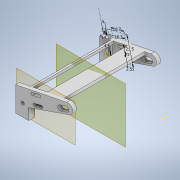
# Autodesk Inventor part: Capping_RotatingArm
Saved by Autodesk Inventor 2022 (Build 260153000, 153)
## iProperties
Created: 2024-05-06
Part Number: Capping_RotatingArm
Material: Generic
Document SubType Name: Modeling
Designer: Gotham City
Density: 1 g/cm^3
Appearance: Default
Author: Gotham City
Autodesk Inventor part; units mm, degrees
ref_plane "YZ Plane" through (0, 0, 0) normal (1, 0, 0) x (0, 1, 0)
ref_plane "XZ Plane" through (0, 0, 0) normal (0, 1, 0) x (-1, 0, 0)
ref_plane "XY Plane" through (0, 0, 0) normal (0, 0, 1) x (1, 0, 0)
sketch "Sketch1" plane through (0, 0, 0) normal (0, 0, 1) x (1, 0, 0)
  line L0 (-13.4159, 40.4526) -> (-44.6613, 29.6117) construction
  circle A0 centre (-45.1029, 22.9379) radius 1.3 projected
  line L1 (-41.8029, 32.9379) -> (-41.8029, 12.9379) projected
  line L2 (-11.7769, 35.7289) -> (-42.4029, 25.1029) construction
  point P0 (0, 0)
sketch "Sketch3" plane through (0, 0, 0) normal (0, 0, 1) x (1, 0, 0)
  line L0 (-41.8029, 32.9379) -> (-41.8029, 12.9379) construction
  line L1 (-41.8029, 12.9379) -> (-50.8029, 12.9379)
  line L2 (-50.8029, 12.9379) -> (-50.8029, 32.9379)
  line L3 (-50.8029, 32.9379) -> (-41.8029, 32.9379)
  line L4 (-41.8029, 32.9379) -> (-41.8029, 12.9379)
  line L5 (-50.8029, 22.9379) -> (-41.8029, 22.9379) construction
  circle A0 centre (-45.1029, 22.9379) radius 1.3 projected
  line L6 (-13.4159, 40.4526) -> (-44.5892, 29.6368)
  line L7 (-44.5892, 29.6368) -> (-41.8029, 21.6064)
  line L8 (-41.8029, 21.6064) -> (-10.6297, 32.4223)
  line L9 (-10.6297, 32.4223) -> (-13.4159, 40.4526)
  line L10 (-13.4159, 40.4526) -> (-41.8029, 21.6064) construction
  line L11 (-44.5892, 29.6368) -> (-10.6297, 32.4223) construction
  line L12 (-42.4029, 25.1029) -> (-11.7769, 35.7289) construction
  line L13 (-13.4159, 40.4526) -> (-44.6613, 29.6117) construction
  circle A1 centre (-11.7769, 35.7289) radius 1.5 construction
  line L14 (-50.8029, 32.9379) -> (-13.4159, 40.4526)
  line L15 (-13.4159, 40.4526) -> (-9.411, 41.2576)
  line L16 (-11.7769, 35.7289) -> (-9.8874, 36.3845) construction
  line L17 (-13.9556, 32.856) -> (-9.2319, 34.495)
  line L18 (-10.543, 38.274) -> (-15.2668, 36.635)
  arc A2 (-9.2319, 34.495) -> (-10.543, 38.274) centre (-9.8874, 36.3845) ccw
  line L19 (-10.6297, 32.4223) -> (-7.3157, 33.5721)
  arc A3 (-7.3157, 33.5721) -> (-9.411, 41.2576) centre (-8.6243, 37.3437) ccw
  arc A4 (-15.2668, 36.635) -> (-13.9556, 32.856) centre (-14.6112, 34.7455) ccw
  point P0 (0, 0)
  point P1 (-27.6094, 31.0295)
  point P2 (-41.8029, 30.6035)
  point P3 (-11.2853, 34.3118)
  point P4 (-12.2686, 37.146)
  point P5 (-10.8322, 36.0567)
  dimension "d0" = 9
  dimension "d1" = 3.5
  dimension "d2" = 0
  dimension "d3" = 3
  dimension "d45" = 4
  dimension "d46" = 2
  dimension "d48" = 7.5
  dimension "d65" = 3
  constraints: 39 end point, 6 parallel, 6 point on circle, 6 tangent, 5 midpoint, 5 point on line, 4 centre point, 3 coincident, 3 perpendicular, 2 collinear, 1 horizontal
  measures "d0" distance of L2.end L3.end
  measures "d1" distance between parallel lines of L8 L12
  measures "d2" distance between parallel lines of L6 L13
  measures "d3" diameter of A1
  measures "d45" distance between parallel lines of L17 L18
  measures "d46" distance of L16.start L16.end
  measures "d65" distance of A4.centre L12.end
extrude "Extrusion1" add sketch "Sketch3" against normal blind 3 contours L1 L2 L3 L4 L6 L7 | L7 L6 L4 | L4 L6 L9 L18 A4 L17 L8 | L14 L6 L4 L3 | L9 L17 A2 L18 L15 A3 L19
ref_plane "Work Plane2" through (0, 0, 32.5) normal (0, 0, 1) x (1, 0, 0)
ref_plane "Work Plane1" through (0, 0, 65) normal (0, 0, 1) x (1, 0, 0)
sketch "Sketch12" plane through (0, 0, -3) normal (0, 0, 1) x (1, 0, 0)
  line L0 (-41.8029, 21.6064) -> (-41.8029, 12.9379) projected
  line L1 (-41.8029, 12.9379) -> (-41.8029, 34.7469)
  line L2 (-41.8029, 34.7469) -> (-40.3029, 35.0484)
  line L3 (-40.3029, 35.0484) -> (-40.3029, 12.9379)
  line L4 (-40.3029, 12.9379) -> (-41.8029, 12.9379)
  line L5 (-9.411, 41.2576) -> (-50.8029, 32.9379) projected
  point P0 (0, 0)
  dimension "d50" = 1.5
  constraints: 8 end point, 2 point on line, 1 collinear, 1 parallel, 1 perpendicular
  measures "d50" distance between parallel lines of L3 L0
extrude "Extrusion9" add sketch "Sketch12" along normal blind 5
thicken "Thicken3" operation add thickness 0.1 both sides no extend neighbours yes toward (1, 0, 0) faces at (-41.8029, 27.4772, 1.3333)
mirror "Mirror1" about plane through (0, 0, 32.5) normal (0, 0, 1) of "Extrusion1", "Extrusion9", "Thicken3"
sketch "Sketch4" plane through (0, 0, 0) normal (0, 0, 1) x (1, 0, 0)
  line L0 (-14.4375, 40.2473) -> (-13.7819, 38.3578)
  line L1 (-13.4159, 40.4526) -> (-44.6613, 29.6117) construction
  line L2 (-13.7819, 38.3578) -> (-27.0084, 33.7687)
  line L3 (-27.0084, 33.7687) -> (-28.2902, 37.4629)
  line L4 (-13.4159, 40.4526) -> (-28.2902, 37.4629)
  line L5 (-50.8029, 32.9379) -> (-9.411, 41.2576) projected
  point P0 (0, 0)
  point P1 (-14.4375, 40.2473)
  point P2 (-14.4375, 40.2473)
  dimension "d8" = 2
  dimension "d9" = 14
  constraints: 6 end point, 2 point on line, 1 perpendicular, 5 other
  measures "d8" distance of point (-14.437, 40.247) L2.start
  measures "d9" distance of L2.start L2.end
extrude "Extrusion2" add sketch "Sketch4" along normal up to surface (65 mm away)
sketch "Sketch10" plane through (-27.0084, 33.7687, 0) normal (0.3277907, -0.9447504, 0) x (0.9447504, 0.3277907, 0)
  line L0 (14, 0) -> (14, 65) construction
  line L1 (0, 0) -> (0, 65) construction
  circle A0 centre (6, 14.5) radius 5
  line L2 (-50.9309, 32.5) -> (44.3132, 32.5) projected
  point P0 (14.4471, 0)
  point P1 (5.5291, 32.5)
  dimension "d25" = 10
  dimension "d28" = 8
  dimension "d68" = 18
  constraints: 1 centre point, 1 point on line
  measures "d25" diameter of A0
  measures "d28" distance from line of A0.centre L0
  measures "d68" vertical distance of A0.centre point (5.529, 32.5)
extrude "Extrusion8" cut sketch "Sketch10" against normal blind 2
draft "FaceDraft1" angle 2.5 pull direction (-0.3277907, 0.9447504, 0) faces at (-17.069, 38.63, 14.0977) fixed edges at (-26.7199, 35.9879, 14.5)
sketch "Sketch16" plane through (0, 0, 0) normal (0, 0, 1) x (1, 0, 0)
  line L0 (-50.8029, 32.9379) -> (-9.411, 41.2576) projected
  line L1 (-39.7029, 35.169) -> (-39.7029, 33.129)
  line L2 (-39.7029, 33.129) -> (-41.7029, 32.727)
  line L3 (-41.7029, 34.767) -> (-41.7029, 12.9379) projected
  line L4 (-41.7029, 34.767) -> (-39.7029, 35.169)
  line L5 (-28.2902, 37.4629) -> (-40.3029, 35.0484) projected
  line L6 (-50.8029, 32.9379) -> (-9.411, 41.2576) projected
  line L7 (-41.7029, 32.727) -> (-41.7029, 34.767)
  point P0 (0, 0)
  dimension "d61" = 2
  dimension "d62" = 2
  constraints: 8 end point, 2 collinear, 2 point on line, 1 parallel, 1 vertical
  measures "d61" distance between parallel lines of L0 L2
  measures "d62" distance between parallel lines of L3 L1
extrude "Extrusion12" add sketch "Sketch16" along normal up to surface (65 mm away)
mirror "Mirror2" about plane through (0, 0, 32.5) normal (0, 0, 1) of "Extrusion8", "FaceDraft1"
sketch "Sketch18" plane through (0, 0, -3) normal (0, 0, -1) x (-1, 0, 0)
  circle A0 centre (32.8063, 27.1171) radius 1 construction
  line L0 (50.8029, 12.9379) -> (50.8029, 32.9379) construction
  circle A1 centre (34.5371, 33.8998) radius 1 construction
  circle A2 centre (45.1029, 22.9379) radius 1.3 construction
  circle A3 centre (45.1029, 22.9379) radius 2.25 construction
  line L1 (28.5428, 20.7228) -> (33.859, 41.5552) construction
  line L2 (33.859, 41.5552) -> (44.2267, 38.9094) construction
  line L3 (44.2267, 38.9094) -> (38.9105, 18.0771) construction
  line L4 (38.9105, 18.0771) -> (28.5428, 20.7228) construction
  line L5 (54.7994, 49.604) -> (46.0227, 15.2108) construction
  line L6 (34.5371, 33.8998) -> (32.8063, 27.1171) construction
  line L7 (31.2009, 31.139) -> (41.5686, 28.4932) construction
  circle A4 centre (48.3029, 34.2571) radius 2.5 construction
  line L8 (32.8063, 27.1171) -> (32.2462, 24.9222) construction
  line L9 (40.3029, 22.1268) -> (7.3157, 33.5721) construction
  line L10 (34.5371, 33.8998) -> (35.0973, 36.0947) construction
  line L11 (28.2902, 37.4629) -> (39.7029, 35.169) construction
  point P0 (0, 0)
  point P1 (33.6717, 30.5085)
  dimension "d69" = 2
  dimension "d71" = 7
  dimension "d78" = 4.5
  dimension "d79" = 14.316
  dimension "d80" = 21.5
  dimension "d82" = 10.7
  dimension "d83" = 18.3
  dimension "d84" = 2.55
  dimension "d85" = 5
  dimension "d86" = 3.5
  constraints: 18 end point, 4 centre point, 4 parallel, 4 point on line, 3 midpoint, 2 collinear, 2 tangent, 1 coincident, 1 equal radius, 1 perpendicular
  measures "d69" diameter of A0
  measures "d71" distance of L6.start L6.end
  measures "d78" diameter of A3
  measures "d79" angle of L0 L5
  measures "d80" distance of L1.start L1.end
  measures "d82" distance of L1.end L2.end
  measures "d83" distance between parallel lines of L1 L5
  measures "d84" distance from line of L1 L6.end
  measures "d85" diameter of A4
  measures "d86" distance from line of L2 A4.centre
sketch "Sketch19" plane through (0, 0, -3) normal (0, 0, -1) x (-1, 0, 0)
  line L0 (35.7131, 26.3753) -> (29.8994, 27.8589) construction
  line L1 (35.4659, 25.4064) -> (29.6522, 26.89)
  line L2 (30.1467, 28.8279) -> (35.9604, 27.3443)
  arc A0 (35.4659, 25.4064) -> (35.9604, 27.3443) centre (35.7131, 26.3753) ccw
  arc A1 (30.1467, 28.8279) -> (29.6522, 26.89) centre (29.8994, 27.8589) ccw
  line L3 (34.5371, 33.8998) -> (32.8063, 27.1171) construction
  line L4 (31.2009, 31.139) -> (41.5686, 28.4932) construction
  line L5 (37.444, 33.158) -> (31.6303, 34.6416) construction
  line L6 (37.6912, 34.1269) -> (31.8776, 35.6105)
  line L7 (31.383, 33.6726) -> (37.1967, 32.189)
  arc A2 (37.1967, 32.189) -> (37.6912, 34.1269) centre (37.444, 33.158) ccw
  arc A3 (31.8776, 35.6105) -> (31.383, 33.6726) centre (31.6303, 34.6416) ccw
  point P0 (0, 0)
  dimension "d87" = 2
  dimension "d88" = 6
  dimension "d53" = 1
  constraints: 16 end point, 8 point on circle, 6 symmetric about line, 4 centre point, 4 tangent, 1 midpoint, 1 parallel, 1 perpendicular, 2 other
  measures "d87" distance between parallel lines of L2 L1
  measures "d88" distance of L0.start L0.end
extrude "Extrusion13" cut sketch "Sketch19" against normal up to surface (71 mm away)
sketch "Sketch15" plane through (-41.8029, 12.9379, 65) normal (-1, 0, 0) x (0, 0, 1)
  line L0 (-49.115, 0) -> (-49.115, 17.165) construction
  line L1 (-49.115, 17.165) -> (-16.115, 17.165) construction
  line L2 (-16.115, 17.165) -> (-16.115, 0) construction
  line L3 (-51.115, 0) -> (-51.115, 19.165)
  line L4 (-51.115, 19.165) -> (-14.115, 19.165)
  line L5 (-14.115, 19.165) -> (-14.115, 0)
  line L6 (-51.115, 0) -> (-14.115, 0)
  line L7 (-65, 0) -> (-49.115, 0) projected
  point P0 (-65, -12.9379)
  dimension "d56" = 2
  constraints: 8 end point, 1 collinear, 1 point on line, 2 other
  measures "d56" distance between parallel lines of L3 L0
ref_plane "Work Plane3" through (0, 0, 32.5) normal (0, 0, 1) x (1, 0, 0)
equation "\"d4\" = d3"
equation "\"d10\" = d3"
body "Solid1"
